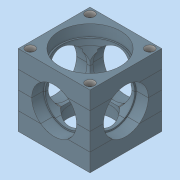
# Autodesk Inventor part: Block
Saved by Autodesk Inventor 2019 (Build 230136000, 136)
## iProperties
Created: 2019-03-27
Part Number: Block
Material: Generisch
Document SubType Name: Modeling
Designer: Martin
Density: 1 g/cm^3
Appearance: Vorgabe
Author: Martin
Autodesk Inventor part; units mm, degrees
ref_plane "YZ Plane" through (0, 0, 0) normal (1, 0, 0) x (0, 1, 0)
ref_plane "XZ Plane" through (0, 0, 0) normal (0, 1, 0) x (-1, 0, 0)
ref_plane "XY Plane" through (0, 0, 0) normal (0, 0, 1) x (1, 0, 0)
sketch "Skizze1" plane through (0, 0, 0) normal (0, 0, 1) x (1, 0, 0)
  line L0 (-60, -60) -> (60, -60)
  line L1 (60, -60) -> (60, 60)
  line L2 (60, 60) -> (-60, 60)
  line L3 (-60, 60) -> (-60, -60)
  line L4 (-60, -60) -> (60, 60) construction
  line L5 (60, -60) -> (-60, 60) construction
  point P0 (0, 0)
  dimension "d0" = 120
  dimension "d1" = 120
  constraints: 12 end point, 2 midpoint, 2 parallel, 1 horizontal, 1 perpendicular
  measures "d0" distance of L2.end L1.end
  measures "d1" distance of L1.end L0.end
extrude "Extrusion1" add sketch "Skizze1" along normal blind 120
sketch "Skizze2" plane through (0, 0, 120) normal (0, 0, 1) x (1, 0, 0)
  circle A0 centre (0, 0) radius 35
  dimension "d4" = 70
  constraints: 1 centre point, 1 coincident
  measures "d4" diameter of A0
extrude "Extrusion2" cut sketch "Skizze2" against normal blind 120
sketch "Skizze3" plane through (60, -60, 0) normal (1, 0, 0) x (0, 0, -1)
  circle A0 centre (-60, 60) radius 35
  line L0 (-120, 0) -> (-120, 120) projected
  line L1 (0, 120) -> (-120, 120) projected
  point P0 (0, 60)
  dimension "d7" = 70
  dimension "d8" = 60
  dimension "d9" = 60
  constraints: 1 centre point
  measures "d7" diameter of A0
  measures "d8" distance from line of A0.centre L0
  measures "d9" distance from line of L1 A0.centre
extrude "Extrusion3" cut sketch "Skizze3" against normal blind 120
sketch "Skizze4" plane through (60, -60, 0) normal (1, 0, 0) x (0, 0, -1)
  circle A0 centre (-60, 60) radius 37.5
  circle A1 centre (-60, 60) radius 35 projected
  point P0 (0, 60)
  dimension "d12" = 75
  constraints: 1 centre point, 1 concentric
  measures "d12" diameter of A0
extrude "Extrusion4" cut sketch "Skizze4" against normal blind 20
sketch "Skizze5" plane through (0, 0, 0) normal (0, 0, -1) x (-1, 0, 0)
  circle A0 centre (0, 0) radius 37.5
  dimension "d15" = 75
  constraints: 1 centre point, 1 coincident
  measures "d15" diameter of A0
extrude "Extrusion5" cut sketch "Skizze5" against normal blind 20
sketch "Skizze6" plane through (-60, -60, 0) normal (-1, 0, 0) x (0, 0, 1)
  circle A0 centre (60, 60) radius 37.5
  circle A1 centre (60, 60) radius 35 projected
  point P0 (0, 60)
  dimension "d18" = 75
  constraints: 1 centre point, 1 concentric
  measures "d18" diameter of A0
extrude "Extrusion6" cut sketch "Skizze6" against normal blind 20
sketch "Skizze7" plane through (0, 0, 120) normal (0, 0, 1) x (1, 0, 0)
  circle A0 centre (0, 0) radius 37.5
  dimension "d21" = 75
  constraints: 1 centre point, 1 coincident
  measures "d21" diameter of A0
extrude "Extrusion7" cut sketch "Skizze7" against normal blind 20
sketch "Skizze8" plane through (-60, 60, 0) normal (0, 1, 0) x (1, 0, 0)
  circle A0 centre (60, -60) radius 51
  line L0 (120, 0) -> (0, 0) projected
  line L1 (0, 0) -> (0, -120) projected
  point P0 (60, 0)
  dimension "d24" = 102
  dimension "d25" = 60
  dimension "d26" = 60
  constraints: 1 centre point
  measures "d24" diameter of A0
  measures "d25" distance from line of L0 A0.centre
  measures "d26" distance from line of A0.centre L1
extrude "Extrusion8" cut sketch "Skizze8" against normal blind 19
sketch "Skizze9" plane through (0, 41, 60) normal (0, 1, 0) x (1, 0, 0)
  line L0 (0, 0) -> (35, 35) projected
  circle A0 centre (0, 0) radius 48.5
  point P0 (0, 60)
  dimension "d29" = 97
  constraints: 1 centre point
  measures "d29" diameter of A0
extrude "Extrusion9" cut sketch "Skizze9" against normal blind 46.75
sketch "Skizze11" plane through (-60, 60, 0) normal (0, 1, 0) x (1, 0, 0)
  line L0 (0, 0) -> (0, -120) projected
  line L1 (120, -120) -> (0, -120) projected
  line L2 (120, 0) -> (0, 0) projected
  line L3 (120, 0) -> (120, -120) projected
  point P0 (60, 0)
  point P1 (10, -110)
  point P2 (10, -10)
  point P3 (110, -110)
  point P4 (110, -10)
  dimension "d36" = 10
  dimension "d37" = 10
  dimension "d38" = 10
  dimension "d39" = 10
  dimension "d40" = 10
  dimension "d48" = 10
  dimension "d49" = 10
  dimension "d50" = 10
  measures "d36" distance from line of point (10, -110) L0
  measures "d37" distance from line of point (10, -110) L1
  measures "d38" distance from line of L0 point (10, -10)
  measures "d39" distance from line of point (10, -10) L2
  measures "d40" distance from line of point (110, -110) L3
  measures "d48" distance from line of point (110, -10) L2
  measures "d49" distance from line of point (110, -10) L3
  measures "d50" distance from line of point (110, -110) L1
hole "Bohrung1" at (-50, 60, 110) at (-50, 60, 10) at (50, 60, 110) at (50, 60, 10) direction (0, -1, 0) diameter 8.5 end through all counterbore diameter 15 counterbore depth 10
thread "Gewinde1" size "M9x1.25" class "6H" standard "ANSI Metric M Profile" length 30
thread "Gewinde2" size "M9x1.25" class "6H" standard "ANSI Metric M Profile" length 30
thread "Gewinde3" size "M9x1.25" class "6H" standard "ANSI Metric M Profile" length 30
thread "Gewinde4" size "M9x1.25" class "6H" standard "ANSI Metric M Profile" length 30
sketch "Skizze12" plane through (-60, -60, 0) normal (0, -1, 0) x (1, 0, 0)
  circle A0 centre (60, 60) radius 37.5
  line L0 (0, 0) -> (120, 0) projected
  line L1 (120, 0) -> (120, 120) projected
  point P0 (60, 0)
  dimension "d59" = 75
  dimension "d60" = 60
  dimension "d61" = 60
  constraints: 1 centre point
  measures "d59" diameter of A0
  measures "d60" distance from line of A0.centre L0
  measures "d61" distance from line of A0.centre L1
extrude "Extrusion11" cut sketch "Skizze12" against normal blind 20
sketch "Skizze13" plane through (0, -40, 60) normal (0, -1, 0) x (1, 0, 0)
  line L0 (35, -35) -> (0, 0) projected
  circle A0 centre (0, 0) radius 35
  point P0 (0, -60)
  point P1 (34.2947, -34.2947)
  dimension "d64" = 70
  constraints: 1 centre point
  measures "d64" diameter of A0
extrude "Extrusion12" cut sketch "Skizze13" against normal blind 34
sketch "Skizze14" plane through (0, 0, 0) normal (0, 0, -1) x (-1, 0, 0)
  line L0 (73, 30) -> (-90, 30)
  line L1 (-90, 30) -> (-90, 29.99)
  line L2 (-90, 29.99) -> (73, 29.99)
  line L3 (73, 29.99) -> (73, 30)
  line L4 (-60, 60) -> (60, 60) projected
  point P0 (0, 0)
  dimension "d67" = 30
  dimension "d68" = 0.01
  constraints: 8 end point, 2 parallel, 1 horizontal, 1 perpendicular
  measures "d67" distance between parallel lines of L4 L0
  measures "d68" distance of L2.end L0.start
extrude "Extrusion13" cut sketch "Skizze14" against normal through all
sketch "Skizze15" plane through (-60, -60, 0) normal (-1, 0, 0) x (0, 0, 1)
  line L0 (138, 60) -> (-47, 60)
  line L1 (-47, 60) -> (-47, 59.99)
  line L2 (-47, 59.99) -> (138, 59.99)
  line L3 (138, 59.99) -> (138, 60)
  line L4 (0, 120) -> (120, 120) projected
  point P0 (0, 60)
  dimension "d71" = 60
  dimension "d72" = 0.01
  constraints: 8 end point, 2 parallel, 1 horizontal, 1 perpendicular
  measures "d71" distance between parallel lines of L4 L0
  measures "d72" distance of L2.end L0.start
extrude "Extrusion14" cut sketch "Skizze15" against normal through all
sketch "Skizze16" plane through (-60, -60, 0) normal (-1, 0, 0) x (0, 0, 1)
  line L0 (144, 30.01) -> (-51, 30.01)
  line L1 (-51, 30.01) -> (-51, 30)
  line L2 (-51, 30) -> (144, 30)
  line L3 (144, 30) -> (144, 30.01)
  line L4 (0, 0) -> (120, 0) projected
  point P0 (0, 60)
  dimension "d75" = 30
  dimension "d76" = 0.01
  constraints: 8 end point, 2 parallel, 1 horizontal, 1 perpendicular
  measures "d75" distance between parallel lines of L4 L2
  measures "d76" distance of L2.end L0.start
extrude "Extrusion15" cut sketch "Skizze16" against normal through all
